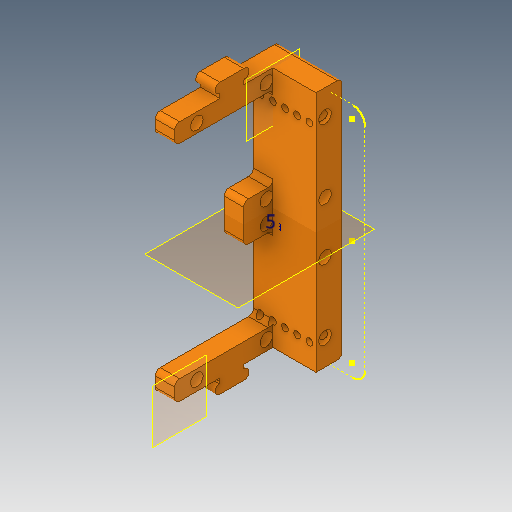
# Autodesk Inventor part: 30_Adapter_neje_to_cube_bd_v3
Saved by Autodesk Inventor 2019.4 (Build 234330000, 330)
## iProperties
Created: 2021-04-09
Part Number: 30_Adapter_neje_to_cube_bd_v3
Material: Generic
Document SubType Name: Modeling
Designer: UC2
Density: 1 g/cm^3
Appearance: Orange
Author: UC2
Autodesk Inventor part; units mm, degrees
ref_plane "YZ Plane" through (0, 0, 0) normal (1, 0, 0) x (0, 1, 0)
ref_plane "XZ Plane" through (0, 0, 0) normal (0, 1, 0) x (-1, 0, 0)
sketch "Skizze1" plane through (0, 0, 0) normal (0, 0, 1) x (1, 0, 0)
  circle A0 centre (-23.32, -39.075) radius 2.355 construction
  circle A1 centre (-23.32, 39.075) radius 2.355 construction
  circle A2 centre (20.82, -6.975) radius 2 construction
  circle A3 centre (20.82, 7.075) radius 2 construction
  line L0 (32.82, 48.575) -> (-32.82, 48.575) construction
  arc A4 (-32.82, 48.575) -> (-34.82, 46.575) centre (-32.82, 46.575) ccw construction
  line L1 (-34.82, 46.575) -> (-34.82, -46.575) construction
  arc A5 (-34.82, -46.575) -> (-32.82, -48.575) centre (-32.82, -46.575) ccw construction
  line L2 (-32.82, -48.575) -> (32.82, -48.575) construction
  arc A6 (32.82, -48.575) -> (34.82, -46.575) centre (32.82, -46.575) ccw construction
  line L3 (34.82, -46.575) -> (34.82, 46.575) construction
  arc A7 (34.82, 46.575) -> (32.82, 48.575) centre (32.82, 46.575) ccw construction
  line L4 (-76.92, -46.575) -> (-35.32, -46.575) construction
  line L5 (-76.92, -40.695) -> (-76.92, -46.575) construction
  line L6 (-42.82, -40.695) -> (-76.92, -40.695) construction
  line L7 (-42.82, -0.875) -> (-42.82, -40.695) construction
  line L8 (-35.32, -0.875) -> (-42.82, -0.875) construction
  line L9 (-35.32, -46.575) -> (-35.32, -0.875) construction
  line L10 (-84.42, -46.575) -> (-76.92, -46.575) construction
  line L11 (-84.42, -0.875) -> (-84.42, -46.575) construction
  line L12 (-42.82, -0.875) -> (-84.42, -0.875) construction
  line L13 (-42.82, -6.755) -> (-42.82, -0.875) construction
  line L14 (-76.92, -6.755) -> (-42.82, -6.755) construction
  line L15 (-76.92, -46.575) -> (-76.92, -6.755) construction
  line L16 (-84.42, 3.425) -> (-76.92, 3.425) construction
  line L17 (-84.42, 49.125) -> (-84.42, 3.425) construction
  line L18 (-42.82, 49.125) -> (-84.42, 49.125) construction
  line L19 (-42.82, 43.245) -> (-42.82, 49.125) construction
  line L20 (-76.92, 43.245) -> (-42.82, 43.245) construction
  line L21 (-76.92, 3.425) -> (-76.92, 43.245) construction
  line L22 (-76.92, 3.425) -> (-35.32, 3.425) construction
  line L23 (-76.92, 9.305) -> (-76.92, 3.425) construction
  line L24 (-42.82, 9.305) -> (-76.92, 9.305) construction
  line L25 (-42.82, 49.125) -> (-42.82, 9.305) construction
  line L26 (-35.32, 49.125) -> (-42.82, 49.125) construction
  line L27 (-35.32, 3.425) -> (-35.32, 49.125) construction
  line L28 (-32.62, -40.5) -> (-32.62, -35.55) construction
  line L29 (-34.82, -40.5) -> (-32.62, -40.5) construction
  line L30 (-34.82, -35.55) -> (-32.62, -35.55) construction
  line L31 (-32.62, -11.9) -> (-32.62, -6.95) construction
  line L32 (-34.82, -11.9) -> (-32.62, -11.9) construction
  line L33 (-34.82, -6.95) -> (-32.62, -6.95) construction
  line L34 (-32.62, 9.5) -> (-32.62, 14.45) construction
  line L35 (-34.82, 9.5) -> (-32.62, 9.5) construction
  line L36 (-34.82, 14.45) -> (-32.62, 14.45) construction
  line L37 (-32.62, 38.1) -> (-32.62, 43.05) construction
  line L38 (-34.82, 38.1) -> (-32.62, 38.1) construction
  line L39 (-34.82, 43.05) -> (-32.62, 43.05) construction
  circle A8 centre (20.82, 7.075) radius 2 construction
  circle A9 centre (20.82, -6.975) radius 2 construction
  line L40 (13.32, -15) -> (17.82, -15) construction
  line L41 (13.32, -9.975) -> (13.32, -15) construction
  line L42 (17.32, -9.975) -> (13.32, -9.975) construction
  line L43 (17.32, -3.975) -> (17.32, -9.975) construction
  line L44 (13.32, -3.975) -> (17.32, -3.975) construction
  line L45 (13.32, 4.075) -> (13.32, -3.975) construction
  line L46 (17.32, 4.075) -> (13.32, 4.075) construction
  line L47 (17.32, 10.075) -> (17.32, 4.075) construction
  line L48 (13.32, 10.075) -> (17.32, 10.075) construction
  line L49 (13.32, 15) -> (13.32, 10.075) construction
  line L50 (17.82, 15) -> (13.32, 15) construction
  line L51 (17.82, 11) -> (17.82, 15) construction
  line L52 (23.82, 11) -> (17.82, 11) construction
  line L53 (23.82, 15) -> (23.82, 11) construction
  line L54 (28.32, 15) -> (23.82, 15) construction
  line L55 (28.32, 10.075) -> (28.32, 15) construction
  line L56 (24.32, 10.075) -> (28.32, 10.075) construction
  line L57 (24.32, 4.075) -> (24.32, 10.075) construction
  line L58 (28.32, 4.075) -> (24.32, 4.075) construction
  line L59 (28.32, -3.975) -> (28.32, 4.075) construction
  line L60 (24.32, -3.975) -> (28.32, -3.975) construction
  line L61 (24.32, -9.975) -> (24.32, -3.975) construction
  line L62 (28.32, -9.975) -> (24.32, -9.975) construction
  line L63 (28.32, -15) -> (28.32, -9.975) construction
  line L64 (23.82, -15) -> (28.32, -15) construction
  line L65 (23.82, -11) -> (23.82, -15) construction
  line L66 (17.82, -11) -> (23.82, -11) construction
  line L67 (17.82, -15) -> (17.82, -11) construction
  line L68 (0.18, 48.575) -> (-34.82, 48.575)
  line L69 (-34.82, 48.575) -> (-34.82, -48.575)
  line L70 (-34.82, -48.575) -> (0.18, -48.575)
  line L71 (5.18, -43.575) -> (5.18, 43.575)
  circle A10 centre (-23.32, 39.075) radius 2.455
  circle A11 centre (-23.32, -39.075) radius 2.255
  arc A12 (0.18, -48.575) -> (5.18, -43.575) centre (0.18, -43.575) ccw
  arc A13 (5.18, 43.575) -> (0.18, 48.575) centre (0.18, 43.575) ccw
  point P0 (0, 0)
  point P1 (5.18, 48.575)
  point P2 (5.18, -48.575)
  dimension "d1" = 0.1
  dimension "d2" = 0.1
  dimension "d8" = 40
  dimension "d9" = 5
  constraints: 24 end point, 9 horizontal, 5 point on line, 4 centre point, 4 point on circle, 4 tangent, 2 parallel, 1 collinear, 1 equal radius, 1 perpendicular, 1 vertical, 9 other
  measures "d1" radial gap between concentric circles of A1 A10
  measures "d2" radial gap between concentric circles of A0 A11
  measures "d8" distance between parallel lines of L71 L69
  measures "d9" radius of A12
extrude "Extrusion1" add sketch "Skizze1" along normal blind 5
sketch "Skizze2" plane through (0, 0, 5) normal (0, 0, 1) x (1, 0, 0)
  circle A0 centre (-23.32, 39.075) radius 2.455 construction
  circle A1 centre (-23.32, -39.075) radius 2.255 construction
  line L0 (0.18, 48.575) -> (-34.82, 48.575) construction
  line L1 (-34.82, 48.575) -> (-34.82, -48.575) construction
  line L2 (-34.82, -48.575) -> (0.18, -48.575) construction
  line L3 (5.18, -43.575) -> (5.18, 43.575) construction
  line L4 (-34.82, 48.575) -> (-29.82, 48.575)
  line L5 (-29.82, 48.575) -> (-29.82, -48.575)
  line L6 (-29.82, -48.575) -> (-34.82, -48.575)
  line L7 (-34.82, -48.575) -> (-34.82, 48.575)
  arc A2 (0.18, -48.575) -> (5.18, -43.575) centre (0.18, -43.575) ccw projected
  arc A3 (5.18, 43.575) -> (0.18, 48.575) centre (0.18, 43.575) ccw projected
  point P0 (0, 0)
  dimension "d5" = 5
  constraints: 8 end point, 2 parallel, 1 horizontal, 1 perpendicular, 1 point on line
  measures "d5" distance between parallel lines of L1 L5
ref_plane "Arbeitsebene1" through (-76.92, -46.575, 102.485) normal (0, 0, 1) x (1, 0, 0)
sketch "Sketch4" plane through (-34.82, -48.575, 0) normal (-1, 0, 0) x (0, 0, 1)
  line L0 (0, 0) -> (0, 97.15) projected
  line L1 (0, 0) -> (5, 0) projected
  line L2 (5, 97.15) -> (5, 0) construction
  line L3 (0, 97.15) -> (5, 97.15) projected
  circle A0 centre (41.935, 4.19) radius 2.475 projected
  circle A1 centre (13.335, 4.19) radius 2.475 projected
  circle A2 centre (13.335, 45.51) radius 2.475 projected
  circle A3 centre (13.335, 54.19) radius 2.475 projected
  circle A4 centre (13.335, 95.51) radius 2.475 projected
  circle A5 centre (41.935, 95.51) radius 2.475 projected
  line L4 (5, 0) -> (51, 0)
  line L5 (51, 0) -> (51, 8)
  line L6 (51, 8) -> (5, 8)
  line L7 (5, 8) -> (5, 0)
  line L8 (5, 8) -> (10.665, 8)
  line L9 (10.665, 8) -> (10.665, 99.5)
  line L10 (10.665, 99.5) -> (5, 99.5)
  line L11 (10.665, 99.5) -> (51, 99.5)
  line L12 (51, 99.5) -> (51, 91.82)
  line L13 (51, 91.82) -> (10.665, 91.82)
  line L14 (10.665, 91.82) -> (10.665, 99.5)
  line L15 (10.665, 41.82) -> (44.605, 41.82) projected
  line L16 (44.605, 57.88) -> (10.665, 57.88) projected
  line L17 (10.665, 41.82) -> (22.665, 41.82)
  line L18 (22.665, 41.82) -> (22.665, 57.88)
  line L19 (22.665, 57.88) -> (10.665, 57.88)
  line L20 (10.665, 57.88) -> (10.665, 41.82)
  line L21 (0, 0) -> (0, 97.15) projected
  line L22 (5, 99.5) -> (0, 99.5)
  line L23 (0, 99.5) -> (0, 0)
  line L24 (0, 0) -> (5, 0)
  line L25 (10.665, 91.82) -> (10.665, 57.88) construction
  line L26 (44.605, 91.82) -> (10.665, 91.82) construction
  line L27 (4.785, 99.7) -> (50.485, 99.7) construction
  line L28 (44.605, 91.82) -> (10.665, 91.82) construction
  circle A6 centre (6.975, 10.55) radius 2.475 projected
  circle A7 centre (6.975, 39.15) radius 2.475 projected
  circle A8 centre (6.975, 60.55) radius 2.475 projected
  circle A9 centre (6.975, 89.15) radius 2.475 projected
  line L29 (5, 97.15) -> (5, 0) projected
  line L30 (5, 40.6416) -> (5, 59.0584)
  line L31 (5, 59.0584) -> (5, 40.6416)
  line L32 (5, 62.0416) -> (5, 87.6584)
  line L33 (5, 90.6416) -> (5, 99.5)
  line L34 (5, 99.5) -> (5, 90.6416)
  line L35 (5, 87.6584) -> (5, 62.0416)
  line L36 (5, 37.6584) -> (5, 12.0416)
  line L37 (5, 9.0584) -> (5, 8)
  line L38 (5, 0) -> (5, 9.0584)
  line L39 (5, 12.0416) -> (5, 37.6584)
  point P0 (0, 48.575)
  dimension "d10" = 46
  dimension "d11" = 8
  dimension "d13" = 91.5
  dimension "d15" = 12
  constraints: 56 end point, 18 parallel, 8 point on circle, 5 horizontal, 5 perpendicular, 4 point on line, 2 coincident, 3 other
  measures "d10" distance of L6.end L5.end
  measures "d11" distance of L5.end L4.end
  measures "d13" distance of L9.end L8.end
  measures "d15" distance of L19.end L18.end
extrude "Extrusion3" add sketch "Sketch4" against normal up to surface (40 mm away) contours L0 L3 L29 A9 A8 A7 A6 L7 L1 | L23 L22 L33 L3 | L7 L6 L5 L4 | L33 L10 L9 L6 L29 A6 A7 A8 A9 | L29 A9 | L11 L12 L13 L9 | L9 L16 L18 L15 picked at (4.8333, 89.15)
fillet "Fillet1" radius 2 12 edges at (-14.82, 43.245, 10.665) (-14.82, 9.305, 22.665) (-14.82, -6.755, 22.665) (-14.82, -40.575, 10.665) (-14.82, -40.575, 51) (-14.82, -48.575, 51) (-14.82, 50.925, 0) (-14.82, -48.575, 0) (-14.82, 43.245, 51) (-14.82, 50.925, 51) (-14.82, 9.305, 10.665) (-14.82, -6.755, 10.665)
sketch "Sketch7" plane through (-34.82, 43.245, 51) normal (-1, 0, 0) x (0, 0, 1)
  circle A0 centre (-37.665, -87.63) radius 2.475 projected
  circle A1 centre (-9.065, -87.63) radius 2.475 projected
  circle A2 centre (-37.665, -46.31) radius 2.475 projected
  circle A3 centre (-37.665, -37.63) radius 2.475 projected
  circle A4 centre (-37.665, 3.69) radius 2.475 projected
  point P0 (-51, -43.245)
sketch "Sketch8" plane through (-34.82, 43.245, 51) normal (-1, 0, 0) x (0, 0, 1)
  circle A0 centre (-44.025, -81.27) radius 2.475 projected
  circle A1 centre (-44.025, -52.67) radius 2.475 projected
  circle A2 centre (-44.025, -31.27) radius 2.475 projected
  circle A3 centre (-44.025, -2.67) radius 2.475 projected
  point P0 (-51, -43.245)
extrude "Extrusion6" cut sketch "Sketch8" against normal blind 6
chamfer "Chamfer1" distance 1 angle 45 18 edges at (-34.82, -44.385, 39.46) (-34.82, -44.385, 10.86) (-34.82, -3.065, 10.86) (-34.82, 5.615, 10.86) (-34.82, 46.935, 10.86) (-34.82, 46.935, 39.46) (-34.82, -9.425, 4.5) (-34.82, -11.7717, 7.7616) (-34.82, -7.0783, 7.7616) (-34.82, 11.975, 4.5) (-34.82, 9.6283, 7.7616) (-34.82, 14.3217, 7.7616) (-34.82, 38.2283, 7.7616) (-34.82, 42.9217, 7.7616) (-34.82, 40.575, 4.5) (-34.82, -38.025, 4.5) (-34.82, -40.3717, 7.7616) (-34.82, -35.6783, 7.7616)
sketch "Sketch10" plane through (0, 0, 0) normal (0, 0, -1) x (-1, 0, 0)
  circle A0 centre (23.32, -39.075) radius 2.355 construction
  circle A1 centre (23.32, 39.075) radius 2.355 construction
  circle A2 centre (-20.82, -6.975) radius 2 projected
  circle A3 centre (-20.82, 7.075) radius 2 projected
  line L0 (-32.82, 48.575) -> (32.82, 48.575) projected
  arc A4 (-32.82, 48.575) -> (-34.82, 46.575) centre (-32.82, 46.575) ccw projected
  line L1 (-34.82, -46.575) -> (-34.82, 46.575) projected
  arc A5 (-34.82, -46.575) -> (-32.82, -48.575) centre (-32.82, -46.575) ccw projected
  line L2 (32.82, -48.575) -> (-32.82, -48.575) projected
  arc A6 (32.82, -48.575) -> (34.82, -46.575) centre (32.82, -46.575) ccw projected
  line L3 (34.82, 46.575) -> (34.82, -46.575) projected
  arc A7 (34.82, 46.575) -> (32.82, 48.575) centre (32.82, 46.575) ccw projected
  circle A8 centre (-3.18, -39.075) radius 1.4
  circle A9 centre (-3.18, 39.075) radius 1.4
  line L4 (-5.18, 48.925) -> (-5.18, -46.575) projected
  point P0 (0, 0)
  dimension "d42" = 2.8
  dimension "d43" = 2.8
  dimension "d44" = 2
  dimension "d45" = 2
  constraints: 2 centre point
  measures "d42" diameter of A8
  measures "d43" diameter of A9
  measures "d44" distance from line of A8.centre L4
  measures "d45" distance from line of A9.centre L4
hole "Hole1" at (3.18, -39.075, 0) at (3.18, 39.075, 0) direction (0, 0, 1) diameter 2.8 end through all
ref_plane "Work Plane4" through (-26.82, -48.575, 49) normal (1, 0, 0) x (0, 0, -1)
ref_plane "Work Plane3" through (-26.82, 41.245, 10.665) normal (1, 0, 0) x (0, 0, -1)
sketch "Sketch12" plane through (-26.82, 41.245, 10.665) normal (1, 0, 0) x (0, 0, -1)
  circle A0 centre (-16.97, 55.89) radius 2.5 projected
  circle A1 centre (4.23, 34.49) radius 2.5 projected
  line L0 (-40.6409, 30.0096) -> (-41.77, 30.0096) projected
  line L1 (-41.77, 30.0096) -> (-41.77, 11.89) projected
  arc A2 (-41.77, 11.89) -> (-39.77, 9.89) centre (-39.77, 11.89) ccw projected
  line L2 (-21.8601, 9.89) -> (-39.77, 9.89) projected
  line L3 (-21.8601, 9.89) -> (-21.8601, 11.0169) projected
  arc A3 (-21.8601, 11.0169) -> (-22.1879, 11.4184) centre (-22.2698, 11.0169) ccw projected
  arc A4 (-21.77, 15.5561) -> (-22.1879, 11.4184) centre (-21.77, 13.4662) ccw projected
  line L4 (-21.77, 15.5561) -> (-11.9714, 15.5561) projected
  arc A5 (-11.429, 11.4483) -> (-11.9714, 15.5561) centre (-11.77, 13.493) ccw projected
  line L5 (-11.429, 11.4483) -> (-11.5497, 11.4178) projected
  arc A6 (-11.5497, 11.4178) -> (-11.8896, 11.0191) centre (-11.4779, 11.0123) ccw projected
  line L6 (-11.8896, 11.0191) -> (-11.8896, 9.89) projected
  line L7 (6.23, 9.89) -> (-11.8896, 9.89) projected
  arc A7 (6.23, 9.89) -> (8.23, 11.89) centre (6.23, 11.89) ccw projected
  line L8 (8.23, 11.89) -> (8.23, 29.89) projected
  line L9 (8.23, 29.89) -> (9.2805, 29.89) projected
  arc A8 (9.7704, 29.49) -> (9.2805, 29.89) centre (9.2805, 29.39) ccw projected
  arc A9 (9.7704, 29.49) -> (13.73, 29.89) centre (11.73, 29.89) ccw projected
  line L10 (13.73, 29.89) -> (13.73, 39.89) projected
  arc A10 (13.73, 39.89) -> (9.7704, 40.29) centre (11.73, 39.89) ccw projected
  arc A11 (9.2805, 39.89) -> (9.7704, 40.29) centre (9.2805, 40.39) ccw projected
  line L11 (9.2805, 39.89) -> (8.23, 39.89) projected
  line L12 (8.23, 39.89) -> (8.23, 57.89) projected
  arc A12 (8.23, 57.89) -> (6.23, 59.89) centre (6.23, 57.89) ccw projected
  line L13 (-11.77, 59.89) -> (6.23, 59.89) projected
  line L14 (-11.77, 59.89) -> (-11.77, 60.9405) projected
  arc A13 (-11.37, 61.4304) -> (-11.77, 60.9405) centre (-11.27, 60.9405) ccw projected
  arc A14 (-11.37, 61.4304) -> (-11.77, 65.39) centre (-11.77, 63.39) ccw projected
  line L15 (-11.77, 65.39) -> (-21.77, 65.39) projected
  arc A15 (-21.77, 65.39) -> (-22.17, 61.4304) centre (-21.77, 63.39) ccw projected
  arc A16 (-21.77, 60.9405) -> (-22.17, 61.4304) centre (-22.27, 60.9405) ccw projected
  line L16 (-21.77, 60.9405) -> (-21.77, 59.89) projected
  line L17 (-39.77, 59.89) -> (-21.77, 59.89) projected
  arc A17 (-39.77, 59.89) -> (-41.77, 57.89) centre (-39.77, 57.89) ccw projected
  line L18 (-41.77, 57.89) -> (-41.77, 39.9801) projected
  line L19 (-41.77, 39.9801) -> (-40.6431, 39.9801) projected
  arc A18 (-40.6431, 39.9801) -> (-40.2416, 40.3079) centre (-40.6431, 40.3898) ccw projected
  arc A19 (-36.1039, 39.89) -> (-40.2416, 40.3079) centre (-38.1938, 39.89) ccw projected
  line L20 (-36.1039, 39.89) -> (-36.1039, 30.0914) projected
  arc A20 (-40.2117, 29.549) -> (-36.1039, 30.0914) centre (-38.167, 29.89) ccw projected
  line L21 (-40.2117, 29.549) -> (-40.2422, 29.6697) projected
  arc A21 (-40.2422, 29.6697) -> (-40.6409, 30.0096) centre (-40.6477, 29.5979) ccw projected
  line L22 (-33.77, 49.89) -> (-33.77, 19.89) projected
  arc A22 (-31.77, 51.89) -> (-33.77, 49.89) centre (-31.77, 49.89) ccw projected
  line L23 (-31.77, 51.89) -> (-1.77, 51.89) projected
  arc A23 (0.23, 49.89) -> (-1.77, 51.89) centre (-1.77, 49.89) ccw projected
  line L24 (0.23, 49.89) -> (0.23, 19.89) projected
  arc A24 (-1.77, 17.89) -> (0.23, 19.89) centre (-1.77, 19.89) ccw projected
  line L25 (-1.77, 17.89) -> (-31.77, 17.89) projected
  arc A25 (-33.77, 19.89) -> (-31.77, 17.89) centre (-31.77, 19.89) ccw projected
  circle A26 centre (-36.77, 14.89) radius 2.425 projected
  circle A27 centre (-37.57, 20.39) radius 2.65 projected
  circle A28 centre (-31.27, 14.09) radius 2.65 projected
  circle A29 centre (3.23, 14.89) radius 2.425 projected
  circle A30 centre (4.03, 20.39) radius 2.65 projected
  circle A31 centre (-2.27, 14.09) radius 2.65 projected
  circle A32 centre (-36.77, 54.89) radius 2.425 projected
  circle A33 centre (-37.57, 49.39) radius 2.65 projected
  circle A34 centre (-31.27, 55.69) radius 2.65 projected
  circle A35 centre (-2.27, 55.69) radius 2.65 projected
  circle A36 centre (4.03, 49.39) radius 2.65 projected
  circle A37 centre (3.23, 54.89) radius 2.425 projected
  arc A38 (-11.5751, 11.5351) -> (-12.0096, 11.02) centre (-11.4779, 11.0123) ccw
  line L26 (-11.5751, 11.5351) -> (-11.4535, 11.5658)
  arc A39 (-11.4535, 11.5658) -> (-11.9655, 15.4361) centre (-11.77, 13.493) ccw
  line L27 (-11.9655, 15.4361) -> (-21.77, 15.4361)
  arc A40 (-21.77, 15.4361) -> (-22.1639, 11.536) centre (-21.77, 13.4662) ccw
  arc A41 (-21.7401, 11.0169) -> (-22.1639, 11.536) centre (-22.2698, 11.0169) ccw
  line L28 (-21.7401, 11.0169) -> (-21.7401, 9.77)
  line L29 (-21.7401, 9.77) -> (-39.77, 9.77)
  arc A42 (-41.89, 11.89) -> (-39.77, 9.77) centre (-39.77, 11.89) ccw
  line L30 (-41.89, 11.89) -> (-41.89, 30.1296)
  line L31 (-41.89, 30.1296) -> (-40.64, 30.1296)
  arc A43 (-40.1249, 29.6951) -> (-40.64, 30.1296) centre (-40.6477, 29.5979) ccw
  line L32 (-40.1249, 29.6951) -> (-40.0942, 29.5735)
  arc A44 (-40.0942, 29.5735) -> (-36.2239, 30.0855) centre (-38.167, 29.89) ccw
  line L33 (-36.2239, 30.0855) -> (-36.2239, 39.89)
  arc A45 (-36.2239, 39.89) -> (-40.124, 40.2839) centre (-38.1938, 39.89) ccw
  arc A46 (-40.6431, 39.8601) -> (-40.124, 40.2839) centre (-40.6431, 40.3898) ccw
  line L34 (-40.6431, 39.8601) -> (-41.89, 39.8601)
  line L35 (-41.89, 39.8601) -> (-41.89, 57.89)
  arc A47 (-39.77, 60.01) -> (-41.89, 57.89) centre (-39.77, 57.89) ccw
  line L36 (-39.77, 60.01) -> (-21.89, 60.01)
  line L37 (-21.89, 60.01) -> (-21.89, 60.9405)
  arc A48 (-21.89, 60.9405) -> (-22.194, 61.3128) centre (-22.27, 60.9405) ccw
  arc A49 (-21.77, 65.51) -> (-22.194, 61.3128) centre (-21.77, 63.39) ccw
  line L38 (-21.77, 65.51) -> (-11.77, 65.51)
  arc A50 (-11.346, 61.3128) -> (-11.77, 65.51) centre (-11.77, 63.39) ccw
  arc A51 (-11.346, 61.3128) -> (-11.65, 60.9405) centre (-11.27, 60.9405) ccw
  line L39 (-11.65, 60.9405) -> (-11.65, 60.01)
  line L40 (-11.65, 60.01) -> (6.23, 60.01)
  arc A52 (8.35, 57.89) -> (6.23, 60.01) centre (6.23, 57.89) ccw
  line L41 (8.35, 57.89) -> (8.35, 40.01)
  line L42 (8.35, 40.01) -> (9.2805, 40.01)
  arc A53 (9.2805, 40.01) -> (9.6528, 40.314) centre (9.2805, 40.39) ccw
  arc A54 (13.85, 39.89) -> (9.6528, 40.314) centre (11.73, 39.89) ccw
  line L43 (13.85, 39.89) -> (13.85, 29.89)
  arc A55 (9.6528, 29.466) -> (13.85, 29.89) centre (11.73, 29.89) ccw
  arc A56 (9.6528, 29.466) -> (9.2805, 29.77) centre (9.2805, 29.39) ccw
  line L44 (9.2805, 29.77) -> (8.35, 29.77)
  line L45 (8.35, 29.77) -> (8.35, 11.89)
  arc A57 (6.23, 9.77) -> (8.35, 11.89) centre (6.23, 11.89) ccw
  line L46 (6.23, 9.77) -> (-12.0096, 9.77)
  line L47 (-12.0096, 9.77) -> (-12.0096, 11.02)
  line L48 (-40.335, 9.68) -> (0, 9.68) projected
  line L49 (-12.0096, 9.77) -> (-12.0096, 9.68)
  line L50 (-21.7401, 9.77) -> (-21.7401, 9.68)
  point P0 (10.665, -41.245)
  dimension "d46" = 0.12
  constraints: 48 end point, 40 point on circle, 20 centre point, 2 perpendicular, 2 point on line, 41 other
  measures "d46" radial gap between concentric circles of A6 A38
extrude "Extrusion9" add sketch "Sketch12" against normal up to surface (8 mm away) contours A38 L47 L49 L48 L50 L28 A41 A40 L27 A39 L26
ref_plane "Work Plane2" through (-34.82, 1.175, 2) normal (0, 1, 0) x (1, 0, 0)
pattern_linear "Rectangular Pattern1" count 8 spacing 5 along (-1, 0, 0) of "Hole1"
sketch "Sketch13" plane through (5.18, 43.245, 51) normal (1, 0, 0) x (0, 0, -1)
  circle A0 centre (9.065, -87.63) radius 2.475 projected
  arc A1 (46, -79.7784) -> (46, -82.7616) centre (44.025, -81.27) ccw projected
  arc A2 (46, -51.1784) -> (46, -54.1616) centre (44.025, -52.67) ccw projected
  arc A3 (46, -29.7784) -> (46, -32.7616) centre (44.025, -31.27) ccw projected
  arc A4 (46, -1.1784) -> (46, -4.1616) centre (44.025, -2.67) ccw projected
  circle A5 centre (44.025, -81.27) radius 2.475
  circle A6 centre (44.025, -52.67) radius 2.475
  circle A7 centre (44.025, -31.27) radius 2.475
  circle A8 centre (44.025, -2.67) radius 2.475
  circle A9 centre (37.925, -87.37) radius 2.45 projected
  circle A10 centre (37.925, 3.73) radius 2.45 projected
  circle A11 centre (9.065, 3.69) radius 2.475 projected
  line L0 (34.1051, -90.5831) -> (41.55, -90.5831)
  line L1 (41.55, -90.5831) -> (41.55, -84.4088)
  line L2 (41.55, -84.4088) -> (34.1051, -84.4088)
  line L3 (34.1051, -84.4088) -> (34.1051, -90.5831)
  line L4 (34.1051, 7.165) -> (41.55, 7.165)
  line L5 (41.55, 7.165) -> (41.55, 0.215)
  line L6 (41.55, 0.215) -> (34.1051, 0.215)
  line L7 (34.1051, 0.215) -> (34.1051, 7.165)
  point P0 (51, -43.245)
  constraints: 16 end point, 4 centre point, 4 coincident, 4 concentric, 4 parallel, 2 horizontal, 2 perpendicular, 2 point on line
extrude "Extrusion10" add sketch "Sketch13" against normal blind 35 contours A0 | A5 A1 | A6 A2 | A7 A3 | A8 A4 | A9 | A10 | A11 | L3 L2 L1 L0 | L4 L5 L6 L7
sketch "Sketch14" plane through (-34.82, 50.925, 51) normal (0, 1, 0) x (1, 0, 0)
  line L0 (1, 40.14) -> (40, 40.14) projected
  line L1 (46.8001, -12.5493) -> (8, -12.5493)
  line L2 (8, -12.5493) -> (8, 40.14)
  line L3 (8, 40.14) -> (46.8001, 40.14)
  line L4 (46.8001, 40.14) -> (46.8001, -12.5493)
  line L5 (0, 49) -> (0, 51) projected
  line L6 (40, 40.335) -> (0, 40.335) construction
  line L7 (0, 40.335) -> (40, 40.335) projected
  line L8 (46.8001, 40.14) -> (8, 40.14)
  line L9 (8, 40.14) -> (8, 40.335)
  line L10 (8, 40.335) -> (46.8001, 40.335)
  line L11 (46.8001, 40.335) -> (46.8001, 40.14)
  line L12 (8, 40.14) -> (46.8001, 40.14)
  line L13 (46.8001, 40.14) -> (46.8001, 45)
  line L14 (46.8001, 45) -> (8, 45)
  line L15 (8, 45) -> (8, 40.14)
  line L16 (40, 51) -> (0, 51) projected
  point P0 (34.82, 51)
  dimension "d54" = 8
  dimension "d57" = 6
  constraints: 24 end point, 6 parallel, 3 horizontal, 3 perpendicular, 2 point on line
  measures "d54" distance between parallel lines of L2 L5
  measures "d57" distance between parallel lines of L14 L16
extrude "Extrusion11" cut sketch "Sketch14" against normal through all contours L9 L7 L10 L11 L3 L0 | L0 L3 L4 L1 L2
mirror "Mirror2" about plane through (-34.82, 1.175, 2) normal (0, 1, 0) of "Extrusion9"
sketch "Sketch15" plane through (-34.82, 50.925, 2) normal (0, 1, 0) x (1, 0, 0)
  line L0 (53.6564, 13.8781) -> (25.752, 13.8781)
  line L1 (25.752, 13.8781) -> (25.752, -21.9876)
  line L2 (25.752, -21.9876) -> (53.6564, -21.9876)
  line L3 (53.6564, -21.9876) -> (53.6564, 13.8781)
  point P0 (34.82, 2)
  constraints: 8 end point, 2 parallel, 1 horizontal, 1 perpendicular
extrude "Extrusion12" cut sketch "Sketch15" against normal through all
sketch "Sketch16" plane through (-34.82, 11.305, 10.665) normal (-1, 0, 0) x (0, 0, 1)
  circle A0 centre (-3.69, 29.27) radius 3.475 projected
  circle A1 centre (-3.69, -20.73) radius 3.475 projected
  circle A2 centre (2.67, 35.63) radius 3.475 projected
  circle A3 centre (2.67, -14.37) radius 3.475 projected
  circle A4 centre (31.27, -55.69) radius 3.475 projected
  arc A5 (40.335, 37.62) -> (38.335, 39.62) centre (38.335, 37.62) ccw projected
  line L0 (21.7401, 39.62) -> (38.335, 39.62) projected
  line L1 (21.7401, 40.9569) -> (21.7401, 39.62) projected
  arc A6 (22.1639, 41.476) -> (21.7401, 40.9569) centre (22.2698, 40.9569) ccw projected
  arc A7 (22.1639, 41.476) -> (21.77, 45.3761) centre (21.77, 43.4062) ccw projected
  line L2 (11.9655, 45.3761) -> (21.77, 45.3761) projected
  arc A8 (11.9655, 45.3761) -> (11.4535, 41.5058) centre (11.77, 43.433) ccw projected
  line L3 (11.5751, 41.4751) -> (11.4535, 41.5058) projected
  arc A9 (12.0096, 40.96) -> (11.5751, 41.4751) centre (11.4779, 40.9523) ccw projected
  line L4 (12.0096, 39.62) -> (12.0096, 40.96) projected
  line L5 (-8.665, 39.62) -> (12.0096, 39.62) projected
  arc A10 (-8.665, 39.62) -> (-10.665, 37.62) centre (-8.665, 37.62) ccw projected
  line L6 (-10.665, -57.88) -> (-10.665, 37.62) projected
  arc A11 (-10.665, -57.88) -> (-8.665, -59.88) centre (-8.665, -57.88) ccw projected
  line L7 (-8.665, -59.88) -> (12.0096, -59.88) projected
  line L8 (12.0096, -59.88) -> (12.0096, -61.22) projected
  arc A12 (11.5751, -61.7351) -> (12.0096, -61.22) centre (11.4779, -61.2123) ccw projected
  line L9 (11.5751, -61.7351) -> (11.4535, -61.7658) projected
  arc A13 (11.4535, -61.7658) -> (11.9655, -65.6361) centre (11.77, -63.693) ccw projected
  line L10 (11.9655, -65.6361) -> (21.77, -65.6361) projected
  arc A14 (21.77, -65.6361) -> (22.1639, -61.736) centre (21.77, -63.6662) ccw projected
  arc A15 (21.7401, -61.2169) -> (22.1639, -61.736) centre (22.2698, -61.2169) ccw projected
  line L11 (21.7401, -61.2169) -> (21.7401, -59.88) projected
  line L12 (21.7401, -59.88) -> (38.335, -59.88) projected
  arc A16 (38.335, -59.88) -> (40.335, -57.88) centre (38.335, -57.88) ccw projected
  line L13 (40.335, -53.88) -> (40.335, -57.88) projected
  arc A17 (40.335, -53.88) -> (38.335, -51.88) centre (38.335, -53.88) ccw projected
  line L14 (2, -51.88) -> (38.335, -51.88) projected
  arc A18 (0, -49.88) -> (2, -51.88) centre (2, -49.88) ccw projected
  line L15 (0, -49.88) -> (0, -20.06) projected
  arc A19 (2, -18.06) -> (0, -20.06) centre (2, -20.06) ccw projected
  line L16 (2, -18.06) -> (10, -18.06) projected
  arc A20 (10, -18.06) -> (12, -16.06) centre (10, -16.06) ccw projected
  line L17 (12, -16.06) -> (12, -4) projected
  arc A21 (12, -4) -> (10, -2) centre (10, -4) ccw projected
  line L18 (10, -2) -> (2, -2) projected
  arc A22 (0, 0) -> (2, -2) centre (2, 0) ccw projected
  line L19 (0, 0) -> (0, 29.94) projected
  arc A23 (2, 31.94) -> (0, 29.94) centre (2, 29.94) ccw projected
  line L20 (38.335, 31.94) -> (2, 31.94) projected
  arc A24 (38.335, 31.94) -> (40.335, 33.94) centre (38.335, 33.94) ccw projected
  line L21 (40.335, 37.62) -> (40.335, 33.94) projected
  circle A25 centre (2.67, -55.69) radius 3.475 projected
  circle A26 centre (2.67, -5.69) radius 3.475 projected
  circle A27 centre (31.27, 35.63) radius 3.475 projected
  circle A28 centre (-3.69, 0.67) radius 3.475 projected
  circle A29 centre (-3.69, -49.33) radius 3.475 projected
  point P0 (-10.665, -11.305)
hole "Hole2" at (-34.82, 46.935, 41.935) at (-34.82, 46.935, 13.335) at (-34.82, 40.575, 6.975) at (-34.82, 11.975, 6.975) at (-34.82, 5.615, 13.335) at (-34.82, -3.065, 13.335) at (-34.82, -9.425, 6.975) at (-34.82, -38.025, 6.975) at (-34.82, -44.385, 13.335) at (-34.82, -44.385, 41.935) direction (1, 0, 0) diameter 5.2 end through all
